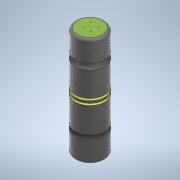
# Autodesk Inventor part: conectorDe2o3pines
Saved by Autodesk Inventor 2020 (Build 240168000, 168)
## iProperties
Created: 2022-02-14
Part Number: conectorDe2o3pines
Material: Genérico
Document SubType Name: Modeling
Designer: DANIEL
Density: 1 g/cm^3
Appearance: Valor por defecto
Author: DANIEL
Autodesk Inventor part; units mm, degrees
ref_plane "XZ Plane" through (0, 0, 0) normal (0, 1, 0) x (-1, 0, 0)
sketch "Boceto1" plane through (0, 0, 0) normal (0, 1, 0) x (-1, 0, 0)
  circle A0 centre (0, 0) radius 12
  dimension "d0" = 24
  constraints: 1 centre point, 1 coincident
  measures "d0" diameter of A0
extrude "Extrusión1" add sketch "Boceto1" along normal mid plane 88
ref_plane "Plano de trabajo1" through (0, 0, 0) normal (0, 1, 0) x (1, 0, 0)
ref_plane "Plano de trabajo2" through (0, 0, 0) normal (1, 0, 0) x (0, 1, 0)
sketch "Boceto2" plane through (0, 0, 0) normal (1, 0, 0) x (0, 1, 0)
  line L0 (-44, 12) -> (-44, -12) projected
  line L1 (44, -12) -> (44, 12) projected
  line L2 (-44, 12) -> (44, 12) projected
  circle A0 centre (1.7, 12) radius 0.75
  line L3 (0, 17.7) -> (0, -16.95) projected
  circle A1 centre (-1.7, 12) radius 0.75
  line L4 (44.17, 0) -> (-44.17, 0) projected
  point P0 (0, 0)
  dimension "d4" = 1.5
  dimension "d5" = 1.7
  dimension "d6" = 1.5
  dimension "d7" = 1.7
  constraints: 2 centre point, 2 point on line
  measures "d4" diameter of A0
  measures "d5" distance from line of L3 A0.centre
  measures "d6" diameter of A1
  measures "d7" distance from line of L3 A1.centre
ref_plane "Plano de trabajo3" through (0, 0, 0) normal (0, 0, 1) x (1, 0, 0)
revolve "Revolución1" cut sketch "Boceto2" angle 360 about axis through (0, 0, 0) along (0, -1, 0) contours A1 L2 | L2 A1 | A0 L2 | L2 A0
sketch "Boceto3" plane through (0, 0, 0) normal (1, 0, 0) x (0, 1, 0)
  line L0 (2.45, 12) -> (44, 12) projected
  circle A0 centre (25, 12) radius 2.5
  circle A1 centre (-25, 10.15) radius 2.5
  line L1 (42.26, 0) -> (-32.71, 0) projected
  point P0 (0, 0)
  dimension "d10" = 5
  dimension "d11" = 25
  dimension "d12" = 5
  dimension "d13" = 25
  constraints: 2 centre point, 1 point on line
  measures "d10" diameter of A0
  measures "d11" horizontal distance of A0.centre point (0, 0)
  measures "d12" diameter of A1
  measures "d13" horizontal distance of point (0, 0) A1.centre
revolve "Revolución2" cut sketch "Boceto3" angle 360 about axis through (0, 0, 0) along (0, -1, 0)
fillet "Empalme1" radius 2 2 edges at (12, 44, 0) (12, -44, 0)
sketch "Boceto4" plane through (0, 44, 0) normal (0, 1, 0) x (1, 0, 0)
  point P0 (0, 0)
  point P1 (0, 0)
  constraints: 1 coincident
